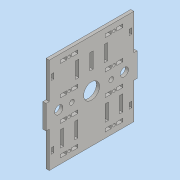
# Autodesk Inventor part: Y-Anchor_Front-Inner
Saved by Autodesk Inventor 2016 SP1 (Build 200210100, 210)
## iProperties
Created: 2015-12-01
Part Number: Y-Anchor_Front-Inner
Material: Generic
Document SubType Name: Modeling
Designer: Mohamed A.
Density: 1 g/cm^3
Appearance: Default
Author: Mohamed A.
Autodesk Inventor part; units mm, degrees
ref_plane "YZ Plane" through (0, 0, 0) normal (1, 0, 0) x (0, 1, 0)
ref_plane "XZ Plane" through (0, 0, 0) normal (0, 1, 0) x (-1, 0, 0)
ref_plane "XY Plane" through (0, 0, 0) normal (0, 0, 1) x (1, 0, 0)
sketch "Sketch1" plane through (0, 0, 0) normal (0, 0, 1) x (1, 0, 0)
  circle A0 centre (0, 0) radius 7.5
  circle A1 centre (18.5, 0) radius 2.25
  circle A2 centre (-18.5, 0) radius 2.25
  circle A3 centre (30.8333, 0) radius 3.9
  circle A4 centre (-30.8333, 0) radius 3.9
  line L0 (-51.1513, 0) -> (71.4472, 0) construction
  line L1 (15.8333, -16.9294) -> (39.8333, -16.9294) construction
  line L2 (39.8333, -16.9294) -> (39.8333, -31.9294)
  line L3 (39.8333, -31.9294) -> (15.8333, -31.9294) construction
  line L4 (15.8333, -31.9294) -> (15.8333, -16.9294) construction
  arc A5 (-21.25, 4.9867) -> (-24, 2.1319) centre (-18.93, 0) ccw construction
  line L5 (-24, -2.1319) -> (-24, 2.1319) construction
  arc A6 (-24, -2.1319) -> (-21.25, -4.9867) centre (-18.93, 0) ccw construction
  line L6 (-10.125, -8.9294) -> (-21.25, -4.9867) construction
  arc A7 (-10.125, -8.9294) -> (10.125, -8.9294) centre (0, 0) ccw construction
  line L7 (21.25, -4.9867) -> (10.125, -8.9294) construction
  arc A8 (21.25, -4.9867) -> (24, -2.1319) centre (18.93, 0) ccw construction
  line L8 (24, 2.1319) -> (24, -2.1319) construction
  arc A9 (24, 2.1319) -> (21.25, 4.9867) centre (18.93, 0) ccw construction
  line L9 (10.125, 8.9294) -> (21.25, 4.9867) construction
  arc A10 (10.125, 8.9294) -> (-10.125, 8.9294) centre (0, 0) ccw construction
  line L10 (-21.25, 4.9867) -> (-10.125, 8.9294) construction
  line L11 (0, 50.1847) -> (0, -53.8877) construction
  line L12 (12.8333, -8.9294) -> (18.4333, -8.9294)
  line L13 (29.3333, -8.9294) -> (29.3333, -11.9294)
  line L14 (29.3333, -11.9294) -> (23.7333, -11.9294)
  line L15 (12.8333, -11.9294) -> (12.8333, -8.9294)
  line L16 (27.8333, -15.5254) -> (27.8333, -35.4643) construction
  line L17 (48.9929, -24.4294) -> (9.7408, -24.4294) construction
  line L18 (21.0833, -5.8226) -> (21.0833, -14.0511) construction
  line L19 (39.8333, 26.6294) -> (39.8333, 27.7794)
  line L20 (39.8333, 31.9294) -> (39.8333, 30.7794)
  line L21 (39.8333, 27.7794) -> (39.8333, 26.6294)
  line L22 (39.8333, 30.7794) -> (39.8333, 31.9294)
  line L23 (42.8333, 11.2324) -> (39.8333, 11.2324)
  line L24 (39.8333, -11.2324) -> (42.8333, -11.2324)
  line L25 (39.8333, -26.6294) -> (39.8333, -27.7794)
  line L26 (39.8333, -31.9294) -> (39.8333, -30.7794)
  line L27 (-39.8333, 44.9294) -> (39.8333, 44.9294)
  line L28 (39.8333, -44.9294) -> (-39.8333, -44.9294)
  line L29 (10.125, -8.9294) -> (-10.125, -8.9294) construction
  line L30 (23.7333, -8.9294) -> (23.7333, -11.9294)
  line L31 (18.4333, -8.9294) -> (18.4333, -11.9294)
  line L32 (23.7333, -8.9294) -> (29.3333, -8.9294)
  line L33 (18.4333, -11.9294) -> (12.8333, -11.9294)
  circle A11 centre (21.0833, -10.4294) radius 1.4
  line L34 (12.8333, -39.9294) -> (18.4333, -39.9294)
  line L35 (29.3333, -39.9294) -> (29.3333, -36.9294)
  line L36 (29.3333, -36.9294) -> (23.7333, -36.9294)
  line L37 (12.8333, -36.9294) -> (12.8333, -39.9294)
  line L38 (23.7333, -39.9294) -> (23.7333, -36.9294)
  line L39 (18.4333, -39.9294) -> (18.4333, -36.9294)
  line L40 (23.7333, -39.9294) -> (29.3333, -39.9294)
  line L41 (18.4333, -36.9294) -> (12.8333, -36.9294)
  circle A12 centre (21.0833, -38.4294) radius 1.4
  line L42 (26.3333, -16.9294) -> (29.3333, -16.9294)
  line L43 (29.3333, -16.9294) -> (29.3333, -31.9294)
  line L44 (29.3333, -31.9294) -> (26.3333, -31.9294)
  line L45 (26.3333, -31.9294) -> (26.3333, -16.9294)
  line L46 (15.8333, -16.9294) -> (12.8333, -16.9294)
  line L47 (12.8333, -16.9294) -> (12.8333, -31.9294)
  line L48 (12.8333, -31.9294) -> (15.8333, -31.9294)
  line L49 (15.8333, -31.9294) -> (15.8333, -16.9294)
  line L50 (-12.8333, -8.9294) -> (-18.4333, -8.9294)
  line L51 (-29.3333, -8.9294) -> (-29.3333, -11.9294)
  line L52 (-29.3333, -11.9294) -> (-23.7333, -11.9294)
  line L53 (-12.8333, -11.9294) -> (-12.8333, -8.9294)
  line L54 (-23.7333, -8.9294) -> (-23.7333, -11.9294)
  line L55 (-18.4333, -8.9294) -> (-18.4333, -11.9294)
  line L56 (-23.7333, -8.9294) -> (-29.3333, -8.9294)
  line L57 (-18.4333, -11.9294) -> (-12.8333, -11.9294)
  circle A13 centre (-21.0833, -10.4294) radius 1.4
  circle A14 centre (-21.0833, -38.4294) radius 1.4
  line L58 (-23.7333, -39.9294) -> (-29.3333, -39.9294)
  line L59 (-23.7333, -39.9294) -> (-23.7333, -36.9294)
  line L60 (-29.3333, -36.9294) -> (-23.7333, -36.9294)
  line L61 (-29.3333, -39.9294) -> (-29.3333, -36.9294)
  line L62 (-12.8333, -39.9294) -> (-18.4333, -39.9294)
  line L63 (-18.4333, -39.9294) -> (-18.4333, -36.9294)
  line L64 (-18.4333, -36.9294) -> (-12.8333, -36.9294)
  line L65 (-12.8333, -36.9294) -> (-12.8333, -39.9294)
  line L66 (-26.3333, -16.9294) -> (-29.3333, -16.9294)
  line L67 (-29.3333, -16.9294) -> (-29.3333, -31.9294)
  line L68 (-29.3333, -31.9294) -> (-26.3333, -31.9294)
  line L69 (-26.3333, -31.9294) -> (-26.3333, -16.9294)
  line L70 (-15.8333, -16.9294) -> (-12.8333, -16.9294)
  line L71 (-12.8333, -16.9294) -> (-12.8333, -31.9294)
  line L72 (-12.8333, -31.9294) -> (-15.8333, -31.9294)
  line L73 (-15.8333, -31.9294) -> (-15.8333, -16.9294)
  line L74 (12.8333, 8.9294) -> (18.4333, 8.9294)
  line L75 (29.3333, 8.9294) -> (29.3333, 11.9294)
  line L76 (29.3333, 11.9294) -> (23.7333, 11.9294)
  line L77 (12.8333, 11.9294) -> (12.8333, 8.9294)
  line L78 (23.7333, 8.9294) -> (23.7333, 11.9294)
  line L79 (18.4333, 8.9294) -> (18.4333, 11.9294)
  line L80 (23.7333, 8.9294) -> (29.3333, 8.9294)
  line L81 (18.4333, 11.9294) -> (12.8333, 11.9294)
  circle A15 centre (21.0833, 10.4294) radius 1.4
  circle A16 centre (21.0833, 38.4294) radius 1.4
  line L82 (23.7333, 39.9294) -> (29.3333, 39.9294)
  line L83 (23.7333, 39.9294) -> (23.7333, 36.9294)
  line L84 (29.3333, 36.9294) -> (23.7333, 36.9294)
  line L85 (29.3333, 39.9294) -> (29.3333, 36.9294)
  line L86 (12.8333, 39.9294) -> (18.4333, 39.9294)
  line L87 (18.4333, 39.9294) -> (18.4333, 36.9294)
  line L88 (18.4333, 36.9294) -> (12.8333, 36.9294)
  line L89 (12.8333, 36.9294) -> (12.8333, 39.9294)
  line L90 (-29.3333, 11.9294) -> (-23.7333, 11.9294)
  line L91 (-29.3333, 8.9294) -> (-29.3333, 11.9294)
  line L92 (-23.7333, 8.9294) -> (-29.3333, 8.9294)
  line L93 (-23.7333, 8.9294) -> (-23.7333, 11.9294)
  circle A17 centre (-21.0833, 10.4294) radius 1.4
  line L94 (-18.4333, 8.9294) -> (-18.4333, 11.9294)
  line L95 (-12.8333, 8.9294) -> (-18.4333, 8.9294)
  line L96 (-12.8333, 11.9294) -> (-12.8333, 8.9294)
  line L97 (-18.4333, 11.9294) -> (-12.8333, 11.9294)
  line L98 (-18.4333, 36.9294) -> (-12.8333, 36.9294)
  line L99 (-12.8333, 36.9294) -> (-12.8333, 39.9294)
  line L100 (-12.8333, 39.9294) -> (-18.4333, 39.9294)
  line L101 (-18.4333, 39.9294) -> (-18.4333, 36.9294)
  circle A18 centre (-21.0833, 38.4294) radius 1.4
  line L102 (-23.7333, 39.9294) -> (-23.7333, 36.9294)
  line L103 (-23.7333, 39.9294) -> (-29.3333, 39.9294)
  line L104 (-29.3333, 39.9294) -> (-29.3333, 36.9294)
  line L105 (-29.3333, 36.9294) -> (-23.7333, 36.9294)
  line L106 (12, 31.9294) -> (-12, 31.9294) construction
  line L107 (-12, 31.9294) -> (-12, 16.9294) construction
  line L108 (-12, 16.9294) -> (12, 16.9294) construction
  line L109 (12, 16.9294) -> (12, 31.9294) construction
  line L110 (-17.778, 24.4294) -> (21.8712, 24.4294) construction
  line L111 (12, 31.9294) -> (15, 31.9294)
  line L112 (15, 31.9294) -> (15, 16.9294)
  line L113 (15, 16.9294) -> (12, 16.9294)
  line L114 (12, 16.9294) -> (12, 31.9294)
  line L115 (-12, 31.9294) -> (-15, 31.9294)
  line L116 (-15, 31.9294) -> (-15, 16.9294)
  line L117 (-15, 16.9294) -> (-12, 16.9294)
  line L118 (-12, 16.9294) -> (-12, 31.9294)
  line L119 (-1.5, 16.9294) -> (1.5, 16.9294)
  line L120 (1.5, 16.9294) -> (1.5, 31.9294)
  line L121 (1.5, 31.9294) -> (-1.5, 31.9294)
  line L122 (-1.5, 31.9294) -> (-1.5, 16.9294)
  line L123 (42.8333, 11.2324) -> (42.8333, -11.2324)
  line L124 (39.8333, 11.2324) -> (39.8333, 44.9294)
  line L125 (39.8333, -11.2324) -> (39.8333, -44.9294)
  line L126 (-42.8333, 11.2324) -> (-39.8333, 11.2324)
  line L127 (-39.8333, -11.2324) -> (-42.8333, -11.2324)
  line L128 (-42.8333, 11.2324) -> (-42.8333, -11.2324)
  line L129 (-39.8333, 11.2324) -> (-39.8333, 44.9294)
  line L130 (-39.8333, -11.2324) -> (-39.8333, -44.9294)
  line L131 (35.4333, -27.3034) -> (37.8333, -27.3034)
  line L132 (37.8333, -27.3034) -> (37.8333, -32.6034)
  line L133 (37.8333, -32.6034) -> (35.4333, -32.6034)
  line L134 (35.4333, -32.6034) -> (35.4333, -27.3034)
  line L135 (-35.4333, -27.3034) -> (-37.8333, -27.3034)
  line L136 (-37.8333, -27.3034) -> (-37.8333, -32.6034)
  line L137 (-37.8333, -32.6034) -> (-35.4333, -32.6034)
  line L138 (-35.4333, -32.6034) -> (-35.4333, -27.3034)
  line L139 (35.4333, 27.3034) -> (37.8333, 27.3034)
  line L140 (37.8333, 27.3034) -> (37.8333, 32.6034)
  line L141 (37.8333, 32.6034) -> (35.4333, 32.6034)
  line L142 (35.4333, 32.6034) -> (35.4333, 27.3034)
  line L143 (-35.4333, 27.3034) -> (-37.8333, 27.3034)
  line L144 (-37.8333, 27.3034) -> (-37.8333, 32.6034)
  line L145 (-37.8333, 32.6034) -> (-35.4333, 32.6034)
  line L146 (-35.4333, 32.6034) -> (-35.4333, 27.3034)
  point P0 (0, 0)
  point P1 (22.8911, -3.8157)
  dimension "d2" = 4.5
  dimension "d3" = 4.5
  dimension "d4" = 7.8
  dimension "d5" = 7.8
  dimension "d61" = 15
  dimension "d62" = 24
  dimension "d63" = 15
  dimension "d64" = 3
  dimension "d79" = 3
  dimension "d85" = 22.4647
  dimension "d90" = 5
  dimension "d92" = 5.3
  dimension "d93" = 2.8
  dimension "d94" = 5
  dimension "d95" = 3
  dimension "d96" = 3
  dimension "d97" = 24
  dimension "d98" = 15
  dimension "d99" = 3
  dimension "d100" = 3
  dimension "d101" = 3
  dimension "d102" = 89.8588
  dimension "d103" = 2.4
  dimension "d104" = 5.3
  dimension "d105" = 5
  dimension "d106" = 85.6667
  dimension "d107" = 12.326
  constraints: 294 end point, 94 symmetric about line, 22 parallel, 19 centre point, 16 horizontal, 15 perpendicular, 13 point on circle, 13 point on line, 9 collinear, 7 vertical, 34 other
  measures "d2" diameter of A1
  measures "d3" diameter of A2
  measures "d4" diameter of A3
  measures "d5" diameter of A4
  measures "d61" diameter of A0
  measures "d62" distance of L2.end L3.end
  measures "d63" distance between parallel lines of L3 L1
  measures "d64" distance of L13.start L13.end
  measures "d79" distance of L23.start L23.end
  measures "d85" distance between parallel lines of L24 L23
  measures "d90" distance between parallel lines of L1 L14
  measures "d92" distance between parallel lines of L31 L30
  measures "d93" diameter of A11
  measures "d94" distance between parallel lines of L28 L40
  measures "d95" distance of L43.end L44.end
  measures "d96" distance of L48.end L47.end
  measures "d97" distance of L108.end L107.end
  measures "d98" distance of L107.end L106.end
  measures "d99" distance of L112.end L113.end
  measures "d100" distance of L117.end L116.end
  measures "d101" distance of L121.end L120.end
  measures "d102" distance between parallel lines of L28 L27
  measures "d103" distance of L132.end L133.end
  measures "d104" distance of L131.end L132.end
  measures "d105" distance between parallel lines of L132 L123
  measures "d106" distance between parallel lines of L128 L123
  measures "d107" distance between parallel lines of L28 L133
extrude "Extrusion1" add sketch "Sketch1" against normal blind 3
body "Solid1"
